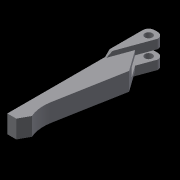
# Autodesk Inventor part: ProximalPhalangeIndex2
Saved by Autodesk Inventor 2015 (Build 190159000, 159)
## iProperties
RuleStatus: InUse
Created: 2014-10-27
Part Number: ProximalPhalangeIndex2
Material: Generic
Document SubType Name: Modeling
Designer: Inventor
Mass: 1.40696 g
Surface Area: 12.5812 cm^2
Volume: 1.40696 cm^3
Density: 1 g/cm^3
Appearance: Default
CX: 8.00 mm
CY: 47.00 mm
CZ: 9.00 mm
Author: Inventor
Autodesk Inventor part; units mm, degrees
ref_plane "YZ Plane" through (0, 0, 0) normal (1, 0, 0) x (0, 1, 0)
ref_plane "XZ Plane" through (0, 0, 0) normal (0, 1, 0) x (-1, 0, 0)
sketch "Base" plane through (0, 0, 0) normal (0, 0, 1) x (1, 0, 0)
  line L0 (0, 0) -> (0, -47)
  line L1 (0, 0) -> (5, 0)
  line L2 (5, 0) -> (5, -2)
  line L3 (3, -7.5) -> (8, -14.5)
  line L4 (8, -14.5) -> (4, -36.5)
  arc A0 (4, -36.5) -> (7, -47) centre (16.1458, -38.7083) ccw
  line L5 (0, -47) -> (7, -47)
  line L6 (5, -2) -> (3, -7.5)
  dimension "d0" = 47
  dimension "d1" = 5
  dimension "d6" = 22
  dimension "d10" = 4
  dimension "d51" = 3
  dimension "d52" = 8
  dimension "d53" = 5.5
  dimension "d54" = 2
  dimension "d55" = 7
  dimension "d112" = 7
  constraints: 14 end point, 2 horizontal, 2 point on circle, 1 centre point, 1 coincident, 1 perpendicular, 1 tangent, 1 vertical
  measures "d0" distance of L0.start L0.end
  measures "d1" distance of L0.start L1.end
  measures "d6" vertical distance of L3.end L4.end
  measures "d10" distance from line of L0 L4.end
  measures "d51" distance from line of L0 L3.start
  measures "d52" distance from line of L0 L3.end
  measures "d53" vertical distance of L2.end L3.start
  measures "d54" distance of L1.end L2.end
  measures "d55" vertical distance of L3.start L3.end
  measures "d112" distance of L0.end L5.end
extrude "BaseFeature" add sketch "Base" along normal blind 9
chamfer "EndChamferFeature" distance 4 angle 45 1 edges at (7, -47, 4.5)
sketch "MountHole" plane through (0, 0, 9) normal (0, 0, 1) x (1, 0, 0)
  circle A0 centre (2.5, -2.5) radius 1.25
  line L0 (5, 0) -> (0, 0) construction
  line L1 (0, 0) -> (0, -47) construction
  dimension "d40" = 2.5
  dimension "d41" = 2.5
  dimension "d42" = 2.5
  constraints: 1 centre point
  measures "d40" diameter of A0
  measures "d41" distance from line of L0 A0.centre
  measures "d42" distance from line of L1 A0.centre
hole "MountHoleFeature" at (2.5, -2.5, 9) direction (0, 0, -1) diameter 2.5 end through all
fillet "EndFilletsFeature" radius 2 2 edges at (0, 0, 4.5) (5, 0, 4.5)
ref_plane "MidPlane" through (0, 0, 4.5) normal (0, 0, 1) x (1, 0, 0)
sketch "MountCut" plane through (0, 0, 4.5) normal (0, 0, 1) x (1, 0, 0)
  line L0 (4.8289, -43.6405) -> (3, -47) projected
  arc A0 (4, -36.5) -> (4.8289, -43.6405) centre (16.1458, -38.7083) ccw projected
  line L1 (4, -36.5) -> (8, -14.5) projected
  line L2 (8, -14.5) -> (3, -7.5) projected
  line L3 (3, -7.5) -> (5, -2) projected
  arc A1 (5, -2) -> (3, 0) centre (3, -2) ccw projected
  line L4 (3, 0) -> (2, 0) projected
  arc A2 (2, 0) -> (0, -2) centre (2, -2) ccw projected
  line L5 (0, -2) -> (0, -47) projected
  circle A3 centre (2.5, -2.5) radius 1.25 projected
  line L6 (3, -7.5) -> (0, -7.5)
  line L7 (8, -14.5) -> (3, -7.5) projected
  line L8 (5.8571, -11.5) -> (0, -11.5)
  line L9 (0, -2) -> (0, -47) projected
  line L10 (0, -47) -> (3, -47) projected
  point P0 (0, -39.1407)
  dimension "d81" = 4
  constraints: 4 end point, 3 point on line, 2 perpendicular
  measures "d81" distance between parallel lines of L8 L6
extrude "MountCutFeature" cut sketch "MountCut" along normal mid plane 3 contours L5 L6 L2 L8 | L5 A2 L4 A1 L3 L6
sketch "LeftTrim" plane through (0, 0, 9) normal (0, 0, 1) x (1, 0, 0)
  line L0 (4.8289, -43.6405) -> (3, -47) projected
  arc A0 (4, -36.5) -> (4.8289, -43.6405) centre (16.1458, -38.7083) ccw projected
  line L1 (4, -36.5) -> (8, -14.5) projected
  line L2 (8, -14.5) -> (3, -7.5) projected
  line L3 (3, -7.5) -> (5, -2) projected
  arc A1 (5, -2) -> (3, 0) centre (3, -2) ccw projected
  line L4 (3, 0) -> (2, 0) projected
  arc A2 (2, 0) -> (0, -2) centre (2, -2) ccw projected
  line L5 (0, -2) -> (0, -47) projected
  circle A3 centre (2.5, -2.5) radius 1.25 projected
  line L6 (3, -7.5) -> (-0.5, -7.5)
  line L7 (0, -47) -> (3, -47) projected
  constraints: 2 end point, 1 horizontal
extrude "LeftTrimFeature" cut sketch "LeftTrim" against normal blind 1.5 contours L0 L7 L5 L6 L2 L1 A0 | L5 A2 L4 A1 L3 L6 | A3
sketch "LeftReinforce" plane through (0, 0, 7.5) normal (0, 0, 1) x (1, 0, 0)
  circle A0 centre (2.5, -2.5) radius 1.25 projected
  line L0 (0, -11.5) -> (0, -2) construction
  line L1 (5.8571, -11.5) -> (0, -11.5) construction
  line L2 (3, -7.5) -> (5.8571, -11.5) construction
  line L3 (5, -2) -> (3, -7.5) projected
  arc A1 (5, -2) -> (3, 0) centre (3, -2) ccw projected
  line L4 (2, 0) -> (3, 0) projected
  arc A2 (2, 0) -> (0, -2) centre (2, -2) ccw projected
  line L5 (0, -11.5) -> (0, -2)
  line L6 (0, -11.5) -> (0, -14.5)
  line L7 (3, -7.5) -> (0.4545, -14.5)
  line L8 (0.4545, -14.5) -> (0, -14.5)
  line L9 (0.4545, -14.5) -> (8, -14.5) construction
  constraints: 10 end point, 3 collinear, 2 horizontal
extrude "LeftReinforceFeature" add sketch "LeftReinforce" along normal blind 1.5
sketch "RightTrim" plane through (0, 0, 0) normal (0, 0, -1) x (-1, 0, 0)
  line L0 (0, -47) -> (0, -14.5) projected
  line L1 (-4.8289, -43.6405) -> (-3, -47) projected
  arc A0 (-4.8289, -43.6405) -> (-4, -36.5) centre (-16.1458, -38.7083) ccw projected
  line L2 (-8, -14.5) -> (-4, -36.5) projected
  line L3 (-3, -7.5) -> (-8, -14.5) projected
  line L4 (-3, -7.5) -> (-0.4545, -14.5) projected
  line L5 (-0.4545, -14.5) -> (0, -14.5) projected
  line L6 (-3, -47) -> (0, -47) projected
extrude "RightTrimFeature" cut sketch "RightTrim" against normal blind 1.5
chamfer "MountSideChamfersFeature" distance 1.5 angle 45 2 edges at (0.2273, -14.5, 9) (0.2273, -14.5, 0)
fillet "MiddleCutBottomFilletFeature" radius 2 1 edges at (0, -11.5, 4.5)
